Autodesk Fusion 360 part; units mm, degrees
(part 2 of 7)
  spline S350 degree 3 poles (139.4271, 55.7466) (139.3722, 56.1473) (139.3138, 56.5474) (139.2519, 56.9471) knots 0 0 0 0 1 1 1 1
  line L94 (27.4293, 60.8238) -> (26.9565, 60.2606)
  line L95 (20.6334, 52.4497) -> (23.1986, 52.6739)
  spline S351 degree 3 poles (30.486, 54.5663) (30.8444, 54.6152) (31.208, 54.5278) (31.505, 54.3214) knots 0 0 0 0 1 1 1 1
  spline S352 degree 3 poles (5.1253, 21.8055) (5.4629, 21.4735) (5.8386, 21.1826) (6.2446, 20.9389) knots 0 0 0 0 1 1 1 1
  spline S353 degree 3 poles (6.2446, 20.9389) (6.6506, 20.695) (7.0841, 20.5001) (7.536, 20.3581) knots 0 0 0 0 1 1 1 1
  spline S354 degree 3 poles (8.9271, 20.0961) (13.5524, 19.7823) (18.173, 19.4041) (22.7877, 18.9618) knots 0 0 0 0 1 1 1 1
  spline S355 degree 3 poles (11.3218, 69.3267) (11.3217, 69.4797) (11.3016, 69.6321) (11.2618, 69.7799) knots 0 0 0 0 1 1 1 1
  spline S356 degree 3 poles (10.8092, 70.5643) (10.7011, 70.6724) (10.5793, 70.7659) (10.4469, 70.8423) knots 0 0 0 0 1 1 1 1
  spline S357 degree 3 poles (4.2406, 22.9109) (4.4908, 22.5088) (4.7878, 22.1378) (5.1253, 21.8055) knots 0 0 0 0 1 1 1 1
  line L96 (9.4976, 59.2549) -> (9.0248, 58.6917)
  spline S358 degree 3 poles (12.9046, 79.647) (12.757, 79.6866) (12.6048, 79.7068) (12.4519, 79.7069) knots 0 0 0 0 1 1 1 1
  line L97 (9.9358, 53.6718) -> (10.9606, 52.8584)
  spline S359 degree 3 poles (36.6117, 17.4425) (41.2123, 16.872) (45.8047, 16.2375) (50.3876, 15.5393) knots 0 0 0 0 1 1 1 1
  line L98 (6.5164, 57.9904) -> (6.9174, 53.4077)
  line L99 (9.5715, 71.0769) -> (9.5715, 71.0769)
  line L100 (10.9606, 52.8584) -> (12.5548, 52.998)
  spline S360 degree 3 poles (11.2618, 69.7799) (11.2223, 69.9274) (11.1636, 70.0692) (11.0872, 70.2015) knots 0 0 0 0 1 1 1 1
  spline S361 degree 3 poles (12.5548, 52.998) (12.9131, 53.0466) (13.2765, 52.959) (13.5733, 52.7525) knots 0 0 0 0 1 1 1 1
  spline S362 degree 3 poles (10.0247, 71.017) (9.8769, 71.0567) (9.7245, 71.0769) (9.5715, 71.0769) knots 0 0 0 0 1 1 1 1
  spline S363 degree 3 poles (7.536, 20.3581) (7.9877, 20.2162) (8.4547, 20.1282) (8.9271, 20.0961) knots 0 0 0 0 1 1 1 1
  line L101 (12.4519, 79.7069) -> (12.4519, 79.7069)
  spline S364 degree 3 poles (15.2828, 57.8989) (15.1809, 57.9845) (15.1178, 58.1074) (15.1076, 58.24) knots 0 0 0 0 1 1 1 1
  line L102 (15.1076, 58.24) -> (15.0203, 59.2363)
  line L103 (32.4104, 61.2595) -> (27.4293, 60.8238)
  spline S365 degree 3 poles (1.0992, 34.3138) (1.3959, 32.5982) (1.7565, 30.8943) (2.1802, 29.2056) knots 0 0 0 0 1 1 1 1
  spline S366 degree 3 poles (8.3344, 70.5643) (8.0061, 70.2361) (7.8217, 69.7909) (7.8217, 69.3267) knots 0 0 0 0 1 1 1 1
  spline S367 degree 3 poles (10.4469, 70.8423) (10.3144, 70.9188) (10.1725, 70.9775) (10.0247, 71.017) knots 0 0 0 0 1 1 1 1
  spline S368 degree 3 poles (13.3268, 79.4723) (13.1943, 79.5487) (13.0524, 79.6074) (12.9046, 79.647) knots 0 0 0 0 1 1 1 1
  spline S369 degree 3 poles (11.0872, 70.2015) (11.0108, 70.3341) (10.9173, 70.4561) (10.8092, 70.5643) knots 0 0 0 0 1 1 1 1
  spline S370 degree 3 poles (13.5733, 52.7525) (13.8701, 52.5461) (14.0786, 52.236) (14.1578, 51.8833) knots 0 0 0 0 1 1 1 1
  line L104 (23.1986, 52.6739) -> (22.7976, 57.2566)
  line L105 (26.9565, 60.2606) -> (26.9983, 59.7825)
  spline S371 degree 3 poles (13.6891, 79.1943) (13.581, 79.3024) (13.4592, 79.3958) (13.3268, 79.4723) knots 0 0 0 0 1 1 1 1
  spline S372 degree 3 poles (8.3344, 68.0895) (8.6625, 67.7614) (9.1075, 67.577) (9.5715, 67.5769) knots 0 0 0 0 1 1 1 1
  line L106 (6.9174, 53.4077) -> (9.9358, 53.6718)
  line L107 (14.1578, 51.8833) -> (14.241, 50.9366)
  spline S373 degree 3 poles (0.092, 44.7003) (0.1305, 42.9597) (0.2339, 41.2211) (0.402, 39.4882) knots 0 0 0 0 1 1 1 1
  spline S374 degree 3 poles (7.8217, 69.3267) (7.8218, 68.8626) (8.0062, 68.4176) (8.3344, 68.0895) knots 0 0 0 0 1 1 1 1
  line L108 (14.241, 50.9366) -> (20.716, 51.5035)
  spline S375 degree 3 poles (3.6391, 24.1925) (3.7883, 23.743) (3.9902, 23.3129) (4.2406, 22.9109) knots 0 0 0 0 1 1 1 1
  spline S376 degree 3 poles (10.8092, 68.0895) (11.1373, 68.4176) (11.3217, 68.8626) (11.3218, 69.3267) knots 0 0 0 0 1 1 1 1
  line L109 (26.9983, 59.7825) -> (24.4481, 59.5593)
  line L110 (20.2324, 57.0323) -> (20.1321, 58.178)
  line L111 (20.1321, 58.178) -> (15.6492, 57.7858)
  line L112 (9.0248, 58.6917) -> (9.0666, 58.2137)
  spline S377 degree 3 poles (2.1802, 29.2056) (2.604, 27.517) (3.0906, 25.8448) (3.6391, 24.1925) knots 0 0 0 0 1 1 1 1
  spline S378 degree 3 poles (0.402, 39.4882) (0.57, 37.7553) (0.8025, 36.0293) (1.0992, 34.3138) knots 0 0 0 0 1 1 1 1
  spline S379 degree 3 poles (9.5715, 71.0769) (9.1075, 71.0768) (8.6625, 70.8925) (8.3344, 70.5643) knots 0 0 0 0 1 1 1 1
  spline S380 degree 3 poles (9.5715, 67.5769) (10.0357, 67.5769) (10.4809, 67.7613) (10.8092, 68.0895) knots 0 0 0 0 1 1 1 1
  line L113 (14.4787, 59.6911) -> (9.4976, 59.2549)
  line L114 (9.0666, 58.2137) -> (6.5164, 57.9904)
  line L115 (22.7976, 57.2566) -> (20.2324, 57.0323)
  spline S381 degree 3 poles (22.7877, 18.9618) (27.4026, 18.5195) (32.011, 18.013) (36.6117, 17.4425) knots 0 0 0 0 1 1 1 1
  line L116 (15.0203, 59.2363) -> (14.4787, 59.6911)
  line L117 (20.716, 51.5035) -> (20.6334, 52.4497)
  spline S382 degree 3 poles (15.6492, 57.7858) (15.5168, 57.7727) (15.3847, 57.8135) (15.2828, 57.8989) knots 0 0 0 0 1 1 1 1
  line L118 (56.1976, 85.7716) -> (51.7033, 85.536)
  spline S383 degree 3 poles (71.8669, 89.3322) (71.7344, 89.4088) (71.5925, 89.4677) (71.4447, 89.5073) knots 0 0 0 0 1 1 1 1
  line L119 (45.607, 87.2191) -> (45.1151, 86.6729)
  spline S384 degree 3 poles (72.5072, 88.6919) (72.4307, 88.8243) (72.3373, 88.946) (72.2292, 89.0541) knots 0 0 0 0 1 1 1 1
  line L120 (64.5051, 83.8436) -> (67.5349, 83.8436)
  line L121 (68.4852, 82.9434) -> (70.0851, 82.9434)
  line L122 (78.0851, 81.6933) -> (80.6602, 81.6933)
  line L123 (80.6602, 81.6933) -> (80.6602, 86.2936)
  spline S385 degree 3 poles (73.5851, 87.4434) (73.4521, 87.4421) (73.3241, 87.4944) (73.2301, 87.5886) knots 0 0 0 0 1 1 1 1
  line L124 (51.1783, 86.0088) -> (51.1255, 87.0077)
  line L125 (67.585, 89.4438) -> (67.0651, 88.9234)
  line L126 (33.0388, 59.8089) -> (32.952, 60.8052)
  spline S386 degree 3 poles (51.7033, 85.536) (51.5707, 85.5278) (51.4403, 85.5732) (51.3416, 85.6621) knots 0 0 0 0 1 1 1 1
  line L127 (45.1399, 86.1933) -> (42.5834, 86.0595)
  line L128 (50.0073, 79.6893) -> (50.0569, 78.7406)
  spline S387 degree 3 poles (72.6818, 88.2697) (72.6423, 88.4174) (72.5836, 88.5594) (72.5072, 88.6919) knots 0 0 0 0 1 1 1 1
  line L129 (67.0651, 88.4438) -> (64.5051, 88.4438)
  spline S388 degree 3 poles (72.2292, 89.0541) (72.1211, 89.1622) (71.9993, 89.2557) (71.8669, 89.3322) knots 0 0 0 0 1 1 1 1
  line L130 (32.0895, 53.4522) -> (32.1722, 52.5055)
  spline S389 degree 3 poles (49.4533, 80.5782) (49.7427, 80.3617) (49.9404, 80.0445) (50.0073, 79.6893) knots 0 0 0 0 1 1 1 1
  spline S390 degree 3 poles (51.3416, 85.6621) (51.2428, 85.7511) (51.1839, 85.876) (51.1783, 86.0088) knots 0 0 0 0 1 1 1 1
  spline S391 degree 3 poles (70.9915, 86.0667) (71.4557, 86.0667) (71.9009, 86.2511) (72.2292, 86.5794) knots 0 0 0 0 1 1 1 1
  line L131 (24.8491, 54.9766) -> (27.8675, 55.2407)
  spline S392 degree 3 poles (69.7544, 89.0541) (69.4262, 88.726) (69.2418, 88.281) (69.2417, 87.817) knots 0 0 0 0 1 1 1 1
  spline S393 degree 3 poles (72.2292, 86.5794) (72.5574, 86.9076) (72.7418, 87.3528) (72.7418, 87.817) knots 0 0 0 0 1 1 1 1
  line L132 (70.3523, 89.4438) -> (67.585, 89.4438)
  line L133 (50.0569, 78.7406) -> (56.548, 79.0806)
  line L134 (56.2575, 84.6229) -> (56.1976, 85.7716)
  spline S394 degree 3 poles (31.505, 54.3214) (31.8018, 54.115) (32.0104, 53.8049) (32.0895, 53.4522) knots 0 0 0 0 1 1 1 1
  line L135 (27.8675, 55.2407) -> (28.8923, 54.4268)
  line L136 (28.8923, 54.4268) -> (30.486, 54.5663)
  line L137 (56.4983, 80.0294) -> (59.0698, 80.1642)
  spline S395 degree 3 poles (71.4447, 89.5073) (71.2969, 89.5469) (71.1445, 89.5669) (70.9915, 89.5668) knots 0 0 0 0 1 1 1 1
  spline S396 degree 3 poles (72.7418, 87.817) (72.7417, 87.9699) (72.7215, 88.1221) (72.6818, 88.2697) knots 0 0 0 0 1 1 1 1
  spline S397 degree 3 poles (33.2145, 59.4678) (33.1125, 59.5533) (33.0491, 59.6762) (33.0388, 59.8089) knots 0 0 0 0 1 1 1 1
  line L138 (45.1151, 86.6729) -> (45.1399, 86.1933)
  line L139 (38.0638, 59.7464) -> (33.5809, 59.3547)
  line L140 (24.4481, 59.5593) -> (24.8491, 54.9766)
  line L141 (51.1255, 87.0077) -> (50.6, 87.4811)
  line L142 (59.0698, 80.1642) -> (58.8289, 84.7578)
  line L143 (45.8504, 81.6241) -> (46.8462, 80.7751)
  line L144 (32.1722, 52.5055) -> (38.6478, 53.0724)
  line L145 (46.8462, 80.7751) -> (48.4441, 80.8588)
  line L146 (70.9915, 89.5668) -> (70.9915, 89.5668)
  line L147 (50.6, 87.4811) -> (45.607, 87.2191)
  spline S398 degree 3 poles (69.2417, 87.817) (69.2417, 87.3528) (69.4261, 86.9076) (69.7544, 86.5794) knots 0 0 0 0 1 1 1 1
  line L148 (64.5051, 88.4438) -> (64.5051, 83.8436)
  line L149 (67.5349, 83.8436) -> (68.4852, 82.9434)
  line L150 (67.0651, 88.9234) -> (67.0651, 88.4438)
  spline S399 degree 3 poles (69.7544, 86.5794) (70.0825, 86.2512) (70.5275, 86.0668) (70.9915, 86.0667) knots 0 0 0 0 1 1 1 1
  line L151 (38.1635, 58.6012) -> (38.0638, 59.7464)
  line L152 (41.1298, 54.2428) -> (40.7288, 58.8255)
  spline S400 degree 3 poles (48.4441, 80.8588) (48.8037, 80.8949) (49.1639, 80.7948) (49.4533, 80.5782) knots 0 0 0 0 1 1 1 1
  line L153 (38.5646, 54.0186) -> (41.1298, 54.2428)
  line L154 (38.6478, 53.0724) -> (38.5646, 54.0186)
  line L155 (58.8289, 84.7578) -> (56.2575, 84.6229)
  spline S401 degree 3 poles (70.9915, 89.5668) (70.5275, 89.5667) (70.0825, 89.3823) (69.7544, 89.0541) knots 0 0 0 0 1 1 1 1
  line L156 (40.7288, 58.8255) -> (38.1635, 58.6012)
  line L157 (42.5834, 86.0595) -> (42.8242, 81.4655)
  line L158 (42.8242, 81.4655) -> (45.8504, 81.6241)
  spline S402 degree 3 poles (33.5809, 59.3547) (33.4485, 59.3416) (33.3165, 59.3824) (33.2145, 59.4678) knots 0 0 0 0 1 1 1 1
  line L159 (32.952, 60.8052) -> (32.4104, 61.2595)
  line L160 (56.548, 79.0806) -> (56.4983, 80.0294)
  line L161 (78.0851, 86.2936) -> (78.0851, 87.4434)
  line L162 (71.5853, 81.6933) -> (71.5853, 80.7435)
  line L163 (78.0851, 80.7435) -> (78.0851, 81.6933)
  line L164 (80.6602, 86.2936) -> (78.0851, 86.2936)
  spline S403 degree 3 poles (71.6313, 89.4438) (71.7125, 89.4125) (71.7912, 89.3752) (71.8669, 89.3322) knots 0 0 0 0 1 1 1 1
  line L165 (73.0849, 88.9435) -> (72.5852, 89.4438)
  line L166 (73.0849, 87.9436) -> (73.0849, 88.9435)
  spline S404 degree 3 poles (71.8669, 89.3322) (71.9993, 89.2557) (72.1211, 89.1622) (72.2292, 89.0541) knots 0 0 0 0 1 1 1 1
  spline S405 degree 3 poles (72.5072, 88.6919) (72.5836, 88.5594) (72.6423, 88.4174) (72.6818, 88.2697) knots 0 0 0 0 1 1 1 1
  spline S406 degree 3 poles (72.2292, 89.0541) (72.3373, 88.946) (72.4307, 88.8243) (72.5072, 88.6919) knots 0 0 0 0 1 1 1 1
  spline S407 degree 3 poles (70.0851, 82.9434) (70.4462, 82.9607) (70.8006, 82.842) (71.0783, 82.6106) knots 0 0 0 0 1 1 1 1
  spline S408 degree 3 poles (72.6818, 88.2697) (72.7215, 88.1221) (72.7417, 87.9699) (72.7418, 87.817) knots 0 0 0 0 1 1 1 1
  spline S409 degree 3 poles (71.0783, 82.6106) (71.3562, 82.3791) (71.5371, 82.0518) (71.5853, 81.6933) knots 0 0 0 0 1 1 1 1
  spline S410 degree 3 poles (72.2292, 86.5794) (71.9009, 86.2511) (71.4557, 86.0667) (70.9915, 86.0667) knots 0 0 0 0 1 1 1 1
  spline S411 degree 3 poles (74.522, 80.7435) (74.4176, 80.5939) (74.3469, 80.4234) (74.3148, 80.2438) knots 0 0 0 0 1 1 1 1
  spline S412 degree 3 poles (69.7544, 89.0541) (69.9248, 89.2237) (70.1283, 89.3563) (70.3523, 89.4438) knots 0 0 0 0 1 1 1 1
  spline S413 degree 3 poles (69.7544, 86.5794) (69.4261, 86.9076) (69.2417, 87.3528) (69.2417, 87.817) knots 0 0 0 0 1 1 1 1
  line L167 (78.0851, 87.4434) -> (73.5851, 87.4434)
  line L168 (72.5852, 89.4438) -> (71.6313, 89.4438)
  spline S414 degree 3 poles (72.7418, 87.817) (72.7418, 87.3528) (72.5574, 86.9076) (72.2292, 86.5794) knots 0 0 0 0 1 1 1 1
  spline S415 degree 3 poles (70.9915, 86.0667) (70.5275, 86.0668) (70.0825, 86.2512) (69.7544, 86.5794) knots 0 0 0 0 1 1 1 1
  line L169 (71.5853, 80.7435) -> (78.0851, 80.7435)
  spline S416 degree 3 poles (73.2301, 87.5886) (73.136, 87.6826) (73.0836, 87.8106) (73.0849, 87.9436) knots 0 0 0 0 1 1 1 1
  spline S417 degree 3 poles (74.3148, 80.2438) (74.3148, 79.9094) (74.4477, 79.5887) (74.6843, 79.3524) knots 0 0 0 0 1 1 1 1
  spline S418 degree 3 poles (75.5752, 78.9834) (75.9094, 78.9834) (76.2298, 79.1162) (76.4661, 79.3524) knots 0 0 0 0 1 1 1 1
  spline S419 degree 3 poles (76.8351, 80.2438) (76.8351, 80.376) (76.8144, 80.5073) (76.7736, 80.6329) knots 0 0 0 0 1 1 1 1
  spline S420 degree 3 poles (69.2417, 87.817) (69.2418, 88.281) (69.4262, 88.726) (69.7544, 89.0541) knots 0 0 0 0 1 1 1 1
  spline S421 degree 3 poles (74.6843, 79.3524) (74.9206, 79.1162) (75.2411, 78.9834) (75.5752, 78.9834) knots 0 0 0 0 1 1 1 1
  line L170 (70.3523, 89.4438) -> (70.3523, 89.4438)
  spline S422 degree 3 poles (76.4661, 79.3524) (76.7025, 79.5888) (76.8352, 79.9095) (76.8351, 80.2438) knots 0 0 0 0 1 1 1 1
  spline S423 degree 3 poles (76.7736, 80.6329) (76.7566, 80.6707) (76.7378, 80.7076) (76.7173, 80.7435) knots 0 0 0 0 1 1 1 1
  spline S424 degree 3 poles (71.5853, 81.6303) (71.5679, 81.6539) (71.5499, 81.6772) (71.5315, 81.7001) knots 0 0 0 0 1 1 1 1
  line L171 (76.7173, 80.7435) -> (74.522, 80.7435)
  spline S425 degree 3 poles (71.5315, 81.7001) (71.4043, 81.8274) (71.261, 81.9376) (71.1052, 82.0277) knots 0 0 0 0 1 1 1 1
  spline S426 degree 3 poles (70.0753, 82.3036) (69.5289, 82.3036) (69.0048, 82.0865) (68.6185, 81.7001) knots 0 0 0 0 1 1 1 1
  spline S427 degree 3 poles (71.1052, 82.0277) (70.9492, 82.1177) (70.7821, 82.1868) (70.6081, 82.2334) knots 0 0 0 0 1 1 1 1
  spline S428 degree 3 poles (68.6185, 81.7001) (68.2322, 81.3139) (68.0151, 80.7901) (68.0149, 80.2438) knots 0 0 0 0 1 1 1 1
  spline S429 degree 3 poles (68.6185, 78.7871) (69.0048, 78.4006) (69.5289, 78.1835) (70.0753, 78.1835) knots 0 0 0 0 1 1 1 1
  line L172 (72.069, 80.7435) -> (71.5853, 80.7435)
  spline S430 degree 3 poles (68.0149, 80.2438) (68.015, 79.6974) (68.2321, 79.1734) (68.6185, 78.7871) knots 0 0 0 0 1 1 1 1
  spline S431 degree 3 poles (63.315, 80.2438) (63.3148, 79.9095) (63.4476, 79.5888) (63.6839, 79.3524) knots 0 0 0 0 1 1 1 1
  spline S432 degree 3 poles (63.6839, 81.1347) (63.4477, 80.8984) (63.315, 80.578) (63.315, 80.2438) knots 0 0 0 0 1 1 1 1
  spline S433 degree 3 poles (64.9645, 81.4417) (64.8387, 81.4827) (64.7072, 81.5036) (64.5748, 81.5037) knots 0 0 0 0 1 1 1 1
  spline S434 degree 3 poles (71.5315, 78.7871) (71.6589, 78.9143) (71.769, 79.0576) (71.8592, 79.2134) knots 0 0 0 0 1 1 1 1
  spline S435 degree 3 poles (72.1351, 80.2438) (72.1336, 80.4125) (72.1114, 80.5803) (72.069, 80.7435) knots 0 0 0 0 1 1 1 1
  spline S436 degree 3 poles (64.5748, 81.5037) (64.2407, 81.5037) (63.9202, 81.371) (63.6839, 81.1347) knots 0 0 0 0 1 1 1 1
  spline S437 degree 3 poles (65.4663, 79.3524) (65.7026, 79.5888) (65.8354, 79.9095) (65.8352, 80.2438) knots 0 0 0 0 1 1 1 1
  spline S438 degree 3 poles (65.7732, 80.6329) (65.7324, 80.7587) (65.6721, 80.8773) (65.5944, 80.9843) knots 0 0 0 0 1 1 1 1
  line L173 (64.5748, 81.5037) -> (64.5748, 81.5037)
  spline S439 degree 3 poles (65.5944, 80.9843) (65.5168, 81.0912) (65.4228, 81.1852) (65.3159, 81.2629) knots 0 0 0 0 1 1 1 1
  spline S440 degree 3 poles (64.4203, 77.3437) (64.0986, 77.3439) (63.8013, 77.1723) (63.6405, 76.8936) knots 0 0 0 0 1 1 1 1
  line L174 (64.4203, 75.5439) -> (65.7303, 75.5439)
  spline S441 degree 3 poles (63.6405, 75.9934) (63.8015, 75.715) (64.0987, 75.5436) (64.4203, 75.5439) knots 0 0 0 0 1 1 1 1
  spline S442 degree 3 poles (63.6405, 76.8936) (63.4797, 76.6151) (63.4797, 76.272) (63.6405, 75.9934) knots 0 0 0 0 1 1 1 1
  spline S443 degree 3 poles (64.5748, 78.9834) (64.9092, 78.9833) (65.2298, 79.116) (65.4663, 79.3524) knots 0 0 0 0 1 1 1 1
  spline S444 degree 3 poles (70.0753, 78.1835) (70.2552, 78.1835) (70.4343, 78.2072) (70.6081, 78.2538) knots 0 0 0 0 1 1 1 1
  spline S445 degree 3 poles (65.7303, 75.5439) (66.0517, 75.5438) (66.3488, 75.7152) (66.5096, 75.9934) knots 0 0 0 0 1 1 1 1
  spline S446 degree 3 poles (70.6081, 82.2334) (70.4343, 82.28) (70.2552, 82.3036) (70.0753, 82.3036) knots 0 0 0 0 1 1 1 1
  spline S447 degree 3 poles (70.6081, 78.2538) (70.7821, 78.3003) (70.9492, 78.3694) (71.1052, 78.4594) knots 0 0 0 0 1 1 1 1
  spline S448 degree 3 poles (72.0648, 79.7105) (72.1115, 79.8845) (72.1351, 80.0637) (72.1351, 80.2438) knots 0 0 0 0 1 1 1 1
  line L175 (71.5853, 80.7435) -> (71.5853, 81.6303)
  spline S449 degree 3 poles (71.1052, 78.4594) (71.261, 78.5496) (71.4043, 78.6597) (71.5315, 78.7871) knots 0 0 0 0 1 1 1 1
  spline S450 degree 3 poles (63.6839, 79.3524) (63.9202, 79.1162) (64.2407, 78.9834) (64.5748, 78.9834) knots 0 0 0 0 1 1 1 1
  spline S451 degree 3 poles (65.8352, 80.2438) (65.8351, 80.376) (65.8142, 80.5073) (65.7732, 80.6329) knots 0 0 0 0 1 1 1 1
  spline S452 degree 3 poles (65.3159, 81.2629) (65.2089, 81.3406) (65.0903, 81.4009) (64.9645, 81.4417) knots 0 0 0 0 1 1 1 1
  spline S453 degree 3 poles (65.7303, 77.3437) (66.0518, 77.3437) (66.3489, 77.1721) (66.5096, 76.8936) knots 0 0 0 0 1 1 1 1
  line L176 (65.7303, 77.3437) -> (64.4203, 77.3437)
  spline S454 degree 3 poles (66.5096, 75.9934) (66.6705, 76.272) (66.6705, 76.6151) (66.5096, 76.8936) knots 0 0 0 0 1 1 1 1
  spline S455 degree 3 poles (66.5096, 76.8936) (66.3489, 77.1721) (66.0518, 77.3437) (65.7303, 77.3437) knots 0 0 0 0 1 1 1 1
  spline S456 degree 3 poles (71.8592, 79.2134) (71.9492, 79.3694) (72.0183, 79.5365) (72.0648, 79.7105) knots 0 0 0 0 1 1 1 1
  line L177 (65.7303, 75.5439) -> (64.4203, 75.5439)
  spline S457 degree 3 poles (63.6405, 76.8936) (63.8013, 77.1723) (64.0986, 77.3439) (64.4203, 77.3437) knots 0 0 0 0 1 1 1 1
  spline S458 degree 3 poles (66.5096, 76.8936) (66.6705, 76.6151) (66.6705, 76.272) (66.5096, 75.9934) knots 0 0 0 0 1 1 1 1
  spline S459 degree 3 poles (64.4203, 75.5439) (64.0987, 75.5436) (63.8015, 75.715) (63.6405, 75.9934) knots 0 0 0 0 1 1 1 1
  line L178 (64.4203, 77.3437) -> (64.4203, 77.3437)
  line L179 (64.4203, 77.3437) -> (65.7303, 77.3437)
  spline S460 degree 3 poles (66.5096, 75.9934) (66.3488, 75.7152) (66.0517, 75.5438) (65.7303, 75.5439) knots 0 0 0 0 1 1 1 1
  spline S461 degree 3 poles (63.6405, 75.9934) (63.4797, 76.272) (63.4797, 76.6151) (63.6405, 76.8936) knots 0 0 0 0 1 1 1 1
  spline S462 degree 3 poles (11.8272, 44.7525) (11.9628, 45.0438) (12.2434, 45.2408) (12.5636, 45.2692) knots 0 0 0 0 1 1 1 1
  spline S463 degree 3 poles (13.3134, 52.2967) (13.1395, 52.3433) (12.9602, 52.367) (12.7801, 52.367) knots 0 0 0 0 1 1 1 1
  spline S464 degree 3 poles (38.9325, 35.4202) (38.9325, 35.0858) (38.7996, 34.7651) (38.563, 34.5288) knots 0 0 0 0 1 1 1 1
  spline S465 degree 3 poles (38.8705, 35.8093) (38.9114, 35.6837) (38.9324, 35.5524) (38.9325, 35.4202) knots 0 0 0 0 1 1 1 1
  line L180 (7.3008, 51.088) -> (7.3008, 51.088)
  spline S466 degree 3 poles (34.1829, 35.474) (34.2296, 35.3) (34.2532, 35.1207) (34.2532, 34.9407) knots 0 0 0 0 1 1 1 1
  spline S467 degree 3 poles (36.4122, 35.4202) (36.4441, 35.5644) (36.5012, 35.7019) (36.5807, 35.8264) knots 0 0 0 0 1 1 1 1
  spline S468 degree 3 poles (34.1829, 34.4074) (34.1363, 34.2335) (34.0672, 34.0666) (33.9772, 33.9107) knots 0 0 0 0 1 1 1 1
  line L181 (86.2118, 38.372) -> (86.2118, 20.7818)
  spline S469 degree 3 poles (8.5612, 49.8276) (8.5611, 49.9599) (8.5402, 50.0914) (8.4992, 50.2172) knots 0 0 0 0 1 1 1 1
  spline S470 degree 3 poles (7.6905, 51.026) (7.5647, 51.067) (7.4332, 51.0879) (7.3008, 51.088) knots 0 0 0 0 1 1 1 1
  spline S471 degree 3 poles (38.7645, 36.0176) (38.8062, 35.9516) (38.8417, 35.8819) (38.8705, 35.8093) knots 0 0 0 0 1 1 1 1
  spline S472 degree 3 poles (6.4099, 48.9367) (6.6462, 48.7004) (6.9667, 48.5677) (7.3008, 48.5677) knots 0 0 0 0 1 1 1 1
  spline S473 degree 3 poles (8.0414, 48.8085) (8.1484, 48.8862) (8.2426, 48.9802) (8.3204, 49.0871) knots 0 0 0 0 1 1 1 1
  spline S474 degree 3 poles (14.1635, 51.8202) (14.0558, 51.923) (13.9373, 52.0138) (13.81, 52.091) knots 0 0 0 0 1 1 1 1
  spline S475 degree 3 poles (8.3204, 49.0871) (8.3981, 49.1941) (8.4584, 49.3127) (8.4992, 49.4385) knots 0 0 0 0 1 1 1 1
  spline S476 degree 3 poles (12.7801, 52.367) (12.2337, 52.3671) (11.7097, 52.1502) (11.3233, 51.7639) knots 0 0 0 0 1 1 1 1
  line L182 (39.3118, 20.7818) -> (39.3118, 36.0657)
  spline S477 degree 3 poles (11.3233, 51.7639) (10.9371, 51.3775) (10.7202, 50.8535) (10.7203, 50.3072) knots 0 0 0 0 1 1 1 1
  spline S478 degree 3 poles (38.563, 34.5288) (38.3267, 34.2925) (38.0063, 34.1598) (37.6721, 34.1598) knots 0 0 0 0 1 1 1 1
  spline S479 degree 3 poles (34.2532, 34.9407) (34.2532, 34.7606) (34.2296, 34.5813) (34.1829, 34.4074) knots 0 0 0 0 1 1 1 1
  line L183 (36.5807, 35.8264) -> (34.1261, 35.6114)
  spline S480 degree 3 poles (7.3008, 51.088) (6.9666, 51.0879) (6.6462, 50.9549) (6.4099, 50.7185) knots 0 0 0 0 1 1 1 1
  spline S481 degree 3 poles (6.4099, 50.7185) (6.1737, 50.4822) (6.041, 50.1617) (6.041, 49.8276) knots 0 0 0 0 1 1 1 1
  spline S482 degree 3 poles (11.9057, 43.8569) (11.7217, 44.12) (11.6917, 44.4613) (11.8272, 44.7525) knots 0 0 0 0 1 1 1 1
  spline S483 degree 3 poles (7.6905, 48.6292) (7.8161, 48.6702) (7.9345, 48.7307) (8.0414, 48.8085) knots 0 0 0 0 1 1 1 1
  spline S484 degree 3 poles (8.0414, 50.8472) (7.9345, 50.9248) (7.8161, 50.9851) (7.6905, 51.026) knots 0 0 0 0 1 1 1 1
  spline S485 degree 3 poles (13.3134, 48.3171) (13.4872, 48.3638) (13.6542, 48.4332) (13.81, 48.5233) knots 0 0 0 0 1 1 1 1
  spline S486 degree 3 poles (6.041, 49.8276) (6.041, 49.4935) (6.1737, 49.173) (6.4099, 48.9367) knots 0 0 0 0 1 1 1 1
  spline S487 degree 3 poles (14.2369, 48.8504) (14.3641, 48.9778) (14.474, 49.1213) (14.564, 49.2772) knots 0 0 0 0 1 1 1 1
  spline S488 degree 3 poles (14.564, 49.2772) (14.6539, 49.4331) (14.7231, 49.6) (14.7696, 49.7739) knots 0 0 0 0 1 1 1 1
  spline S489 degree 3 poles (12.7801, 48.2473) (12.9601, 48.2472) (13.1394, 48.2706) (13.3134, 48.3171) knots 0 0 0 0 1 1 1 1
  line L184 (52.0955, 38.372) -> (86.2118, 38.372)
  spline S490 degree 3 poles (52.0707, 38.8407) (52.1203, 38.6894) (52.1288, 38.5277) (52.0955, 38.372) knots 0 0 0 0 1 1 1 1
  spline S491 degree 3 poles (14.7696, 49.7739) (14.8163, 49.9478) (14.8399, 50.1271) (14.8399, 50.3072) knots 0 0 0 0 1 1 1 1
  line L185 (39.3118, 36.0657) -> (38.7645, 36.0176)
  spline S492 degree 3 poles (37.6721, 34.1598) (37.338, 34.1598) (37.0175, 34.2925) (36.7812, 34.5288) knots 0 0 0 0 1 1 1 1
  line L186 (12.5636, 45.2692) -> (13.8684, 45.3834)
  spline S493 degree 3 poles (7.3008, 48.5677) (7.4331, 48.5676) (7.5646, 48.5884) (7.6905, 48.6292) knots 0 0 0 0 1 1 1 1
  spline S494 degree 3 poles (34.1261, 35.6114) (34.1467, 35.5663) (34.1656, 35.5204) (34.1829, 35.474) knots 0 0 0 0 1 1 1 1
  spline S495 degree 3 poles (8.4992, 50.2172) (8.4584, 50.3429) (8.398, 50.4613) (8.3204, 50.5681) knots 0 0 0 0 1 1 1 1
  line L187 (86.2118, 20.7818) -> (39.3118, 20.7818)
  spline S496 degree 3 poles (8.3204, 50.5681) (8.2426, 50.6752) (8.1485, 50.7694) (8.0414, 50.8472) knots 0 0 0 0 1 1 1 1
  spline S497 degree 3 poles (11.3233, 48.8504) (11.7097, 48.4642) (12.2337, 48.2472) (12.7801, 48.2473) knots 0 0 0 0 1 1 1 1
  line L188 (13.9469, 45.3865) -> (13.9469, 45.3865)
  spline S498 degree 3 poles (13.81, 52.091) (13.6542, 52.181) (13.4872, 52.2501) (13.3134, 52.2967) knots 0 0 0 0 1 1 1 1
  spline S499 degree 3 poles (14.8399, 50.3072) (14.8399, 50.4872) (14.8163, 50.6665) (14.7696, 50.8405) knots 0 0 0 0 1 1 1 1
  spline S500 degree 3 poles (10.7203, 50.3072) (10.7202, 49.7608) (10.9371, 49.2368) (11.3233, 48.8504) knots 0 0 0 0 1 1 1 1
  spline S501 degree 3 poles (36.7812, 34.5288) (36.5448, 34.7652) (36.4121, 35.0859) (36.4122, 35.4202) knots 0 0 0 0 1 1 1 1
  spline S502 degree 3 poles (13.81, 48.5233) (13.966, 48.6132) (14.1095, 48.7232) (14.2369, 48.8504) knots 0 0 0 0 1 1 1 1
  spline S503 degree 3 poles (8.4992, 49.4385) (8.5402, 49.5641) (8.5611, 49.6954) (8.5612, 49.8276) knots 0 0 0 0 1 1 1 1
  spline S504 degree 3 poles (13.8684, 45.3834) (13.8945, 45.3856) (13.9207, 45.3866) (13.9469, 45.3865) knots 0 0 0 0 1 1 1 1
  spline S505 degree 3 poles (54.0664, 60.5825) (53.8302, 60.8188) (53.6975, 61.1393) (53.6975, 61.4734) knots 0 0 0 0 1 1 1 1
  spline S506 degree 3 poles (43.1286, 59.9872) (43.0811, 59.7425) (42.9933, 59.5075) (42.8687, 59.2916) knots 0 0 0 0 1 1 1 1
  spline S507 degree 3 poles (34.9307, 52.3551) (34.9625, 52.4995) (35.0196, 52.6372) (35.0991, 52.7618) knots 0 0 0 0 1 1 1 1
  spline S508 degree 3 poles (41.8967, 62.4439) (42.0484, 62.3707) (42.1914, 62.2808) (42.323, 62.1757) knots 0 0 0 0 1 1 1 1
  spline S509 degree 3 poles (32.7014, 52.4088) (32.7479, 52.2351) (32.7716, 52.056) (32.7716, 51.8761) knots 0 0 0 0 1 1 1 1
  spline S510 degree 3 poles (32.6445, 52.5468) (32.6651, 52.5015) (32.6841, 52.4555) (32.7014, 52.4088) knots 0 0 0 0 1 1 1 1
  spline S511 degree 3 poles (35.2996, 51.4642) (35.0634, 51.7005) (34.9307, 52.021) (34.9307, 52.3551) knots 0 0 0 0 1 1 1 1
  spline S512 degree 3 poles (42.6795, 61.8196) (42.7768, 61.6971) (42.8609, 61.5648) (42.9307, 61.4248) knots 0 0 0 0 1 1 1 1
  spline S513 degree 3 poles (32.4957, 50.8461) (32.4056, 50.6901) (32.2955, 50.5466) (32.1681, 50.4193) knots 0 0 0 0 1 1 1 1
  spline S514 degree 3 poles (54.9574, 60.2135) (54.6232, 60.2135) (54.3027, 60.3462) (54.0664, 60.5825) knots 0 0 0 0 1 1 1 1
  spline S515 degree 3 poles (32.7014, 51.3428) (32.6548, 51.1689) (32.5856, 51.002) (32.4957, 50.8461) knots 0 0 0 0 1 1 1 1
  spline S516 degree 3 poles (42.8687, 59.2916) (42.6713, 58.9498) (42.3874, 58.6658) (42.0455, 58.4684) knots 0 0 0 0 1 1 1 1
  spline S517 degree 3 poles (44.8634, 61.7886) (45.0997, 61.5523) (45.2324, 61.2319) (45.2324, 60.8977) knots 0 0 0 0 1 1 1 1
  spline S518 degree 3 poles (30.133, 34.9407) (30.1331, 35.4871) (30.3502, 36.0111) (30.7366, 36.3974) knots 0 0 0 0 1 1 1 1
  spline S519 degree 3 poles (43.9725, 62.1576) (44.3066, 62.1576) (44.6271, 62.0249) (44.8634, 61.7886) knots 0 0 0 0 1 1 1 1
  spline S520 degree 3 poles (43.9725, 59.6373) (43.6573, 59.6443) (43.3562, 59.7691) (43.1286, 59.9872) knots 0 0 0 0 1 1 1 1
  spline S521 degree 3 poles (36.1905, 51.0952) (35.8564, 51.0952) (35.5359, 51.2279) (35.2996, 51.4642) knots 0 0 0 0 1 1 1 1
  spline S522 degree 3 poles (37.0814, 51.4642) (36.8451, 51.2279) (36.5247, 51.0952) (36.1905, 51.0952) knots 0 0 0 0 1 1 1 1
  line L189 (38.6478, 53.0724) -> (37.283, 52.953)
  spline S523 degree 3 poles (33.6496, 33.4839) (33.5224, 33.3567) (33.3791, 33.2467) (33.2233, 33.1568) knots 0 0 0 0 1 1 1 1
  spline S524 degree 3 poles (54.0664, 62.3643) (54.3027, 62.6006) (54.6232, 62.7333) (54.9574, 62.7333) knots 0 0 0 0 1 1 1 1
  spline S525 degree 3 poles (42.0455, 58.4684) (41.7035, 58.2708) (41.3155, 58.1667) (40.9205, 58.1666) knots 0 0 0 0 1 1 1 1
  spline S526 degree 3 poles (32.1681, 50.4193) (32.0409, 50.2919) (31.8975, 50.1818) (31.7417, 50.0917) knots 0 0 0 0 1 1 1 1
  spline S527 degree 3 poles (31.7417, 50.0917) (31.5857, 50.0017) (31.4186, 49.9325) (31.2446, 49.886) knots 0 0 0 0 1 1 1 1
  spline S528 degree 3 poles (40.9205, 62.6666) (41.0888, 62.6666) (41.2566, 62.6477) (41.4207, 62.6103) knots 0 0 0 0 1 1 1 1
  spline S529 degree 3 poles (31.2446, 49.886) (31.0708, 49.8394) (30.8917, 49.8158) (30.7118, 49.8157) knots 0 0 0 0 1 1 1 1
  spline S530 degree 3 poles (29.2551, 50.4193) (28.8686, 50.8056) (28.6515, 51.3296) (28.6515, 51.8761) knots 0 0 0 0 1 1 1 1
  spline S531 degree 3 poles (29.2551, 53.3323) (29.6414, 53.7187) (30.1654, 53.9359) (30.7118, 53.9359) knots 0 0 0 0 1 1 1 1
  spline S532 degree 3 poles (31.2446, 53.8656) (31.4186, 53.8191) (31.5857, 53.7499) (31.7417, 53.6599) knots 0 0 0 0 1 1 1 1
  spline S533 degree 3 poles (45.2324, 60.8977) (45.2324, 60.5636) (45.0997, 60.2431) (44.8634, 60.0068) knots 0 0 0 0 1 1 1 1
  spline S534 degree 3 poles (37.283, 52.953) (37.3247, 52.887) (37.3601, 52.8173) (37.3889, 52.7447) knots 0 0 0 0 1 1 1 1
  spline S535 degree 3 poles (32.7262, 32.9506) (32.5524, 32.9042) (32.3733, 32.8807) (32.1934, 32.8808) knots 0 0 0 0 1 1 1 1
  line L190 (32.952, 60.8052) -> (33.0388, 59.8089)
  spline S536 degree 3 poles (31.7417, 53.6599) (31.869, 53.5825) (31.9875, 53.4916) (32.0952, 53.3886) knots 0 0 0 0 1 1 1 1
  spline S537 degree 3 poles (32.7262, 36.9302) (32.9001, 36.8837) (33.0673, 36.8145) (33.2233, 36.7245) knots 0 0 0 0 1 1 1 1
  line L191 (54.9574, 62.7333) -> (54.9574, 62.7333)
  spline S538 degree 3 poles (33.2233, 36.7245) (33.3506, 36.6471) (33.4691, 36.5562) (33.5768, 36.4532) knots 0 0 0 0 1 1 1 1
  line L192 (33.5768, 36.4532) -> (33.5711, 36.5168)
  spline S539 degree 3 poles (42.9307, 61.4248) (42.9616, 61.5532) (43.0125, 61.676) (43.0816, 61.7886) knots 0 0 0 0 1 1 1 1
  spline S540 degree 3 poles (44.8634, 60.0068) (44.6272, 59.7704) (44.3067, 59.6375) (43.9725, 59.6373) knots 0 0 0 0 1 1 1 1
  line L193 (40.783, 58.2033) -> (41.1298, 54.2428)
  line L194 (41.1298, 54.2428) -> (38.5646, 54.0186)
  spline S541 degree 3 poles (37.3889, 52.7447) (37.4297, 52.6189) (37.4505, 52.4874) (37.4504, 52.3551) knots 0 0 0 0 1 1 1 1
  spline S542 degree 3 poles (32.7716, 51.8761) (32.7716, 51.696) (32.748, 51.5167) (32.7014, 51.3428) knots 0 0 0 0 1 1 1 1
  spline S543 degree 3 poles (30.7366, 33.4839) (30.3502, 33.8702) (30.1331, 34.3942) (30.133, 34.9407) knots 0 0 0 0 1 1 1 1
  spline S544 degree 3 poles (42.323, 62.1757) (42.4548, 62.0707) (42.5744, 61.9513) (42.6795, 61.8196) knots 0 0 0 0 1 1 1 1
  spline S545 degree 3 poles (32.1934, 37.0005) (32.3733, 37.0004) (32.5524, 36.9768) (32.7262, 36.9302) knots 0 0 0 0 1 1 1 1
  spline S546 degree 3 poles (33.2233, 33.1568) (33.0673, 33.0666) (32.9002, 32.9973) (32.7262, 32.9506) knots 0 0 0 0 1 1 1 1
  spline S547 degree 3 poles (32.1934, 32.8808) (31.647, 32.8807) (31.123, 33.0977) (30.7366, 33.4839) knots 0 0 0 0 1 1 1 1
  spline S548 degree 3 poles (40.9205, 58.1666) (40.8743, 58.1774) (40.8284, 58.1896) (40.783, 58.2033) knots 0 0 0 0 1 1 1 1
  line L195 (35.0991, 52.7618) -> (32.6445, 52.5468)
  spline S549 degree 3 poles (28.6515, 51.8761) (28.6516, 52.4223) (28.8687, 52.9461) (29.2551, 53.3323) knots 0 0 0 0 1 1 1 1
  spline S550 degree 3 poles (30.7118, 49.8157) (30.1654, 49.8157) (29.6414, 50.0329) (29.2551, 50.4193) knots 0 0 0 0 1 1 1 1
  spline S551 degree 3 poles (33.9772, 33.9107) (33.8872, 33.7548) (33.777, 33.6112) (33.6496, 33.4839) knots 0 0 0 0 1 1 1 1
  line L196 (32.0952, 53.3886) -> (32.0895, 53.4522)
  spline S552 degree 3 poles (43.0816, 61.7886) (43.3179, 62.0249) (43.6384, 62.1576) (43.9725, 62.1576) knots 0 0 0 0 1 1 1 1
  spline S553 degree 3 poles (37.4504, 52.3551) (37.4504, 52.021) (37.3177, 51.7005) (37.0814, 51.4642) knots 0 0 0 0 1 1 1 1
  line L197 (32.4104, 61.2595) -> (32.952, 60.8052)
  line L198 (38.5646, 54.0186) -> (38.6478, 53.0724)
  spline S554 degree 3 poles (30.7118, 53.9359) (30.8917, 53.9358) (31.0708, 53.9122) (31.2446, 53.8656) knots 0 0 0 0 1 1 1 1
  spline S555 degree 3 poles (32.0895, 53.4522) (32.0104, 53.8049) (31.8018, 54.115) (31.505, 54.3214) knots 0 0 0 0 1 1 1 1
  spline S556 degree 3 poles (41.4207, 62.6103) (41.5851, 62.5728) (41.7447, 62.517) (41.8967, 62.4439) knots 0 0 0 0 1 1 1 1
  spline S557 degree 3 poles (30.7366, 36.3974) (31.123, 36.7837) (31.647, 37.0006) (32.1934, 37.0005) knots 0 0 0 0 1 1 1 1
  spline S558 degree 3 poles (53.6975, 61.4734) (53.6975, 61.8075) (53.8302, 62.128) (54.0664, 62.3643) knots 0 0 0 0 1 1 1 1
  line L199 (20.716, 51.5035) -> (19.3513, 51.3841)
  line L200 (24.8491, 54.9766) -> (24.4481, 59.5593)
  line L201 (33.5809, 59.3547) -> (38.0638, 59.7464)
  spline S559 degree 3 poles (55.6979, 62.4925) (55.8049, 62.4148) (55.8991, 62.3208) (55.9769, 62.2139) knots 0 0 0 0 1 1 1 1
  line L202 (20.1321, 58.178) -> (20.2324, 57.0323)
  spline S560 degree 3 poles (19.4577, 51.1758) (19.4985, 51.0502) (19.5192, 50.9188) (19.5192, 50.7867) knots 0 0 0 0 1 1 1 1
  line L203 (24.4481, 59.5593) -> (26.9983, 59.7825)
  spline S561 degree 3 poles (33.0388, 59.8089) (33.0491, 59.6762) (33.1125, 59.5533) (33.2145, 59.4678) knots 0 0 0 0 1 1 1 1
  line L204 (20.2324, 57.0323) -> (22.7976, 57.2566)
  spline S562 degree 3 poles (14.8399, 50.3072) (14.8399, 50.1271) (14.8163, 49.9478) (14.7696, 49.7739) knots 0 0 0 0 1 1 1 1
  line L205 (27.8675, 55.2407) -> (24.8491, 54.9766)
  spline S563 degree 3 poles (39.5418, 58.7216) (39.319, 58.8758) (39.1259, 59.0689) (38.9718, 59.2916) knots 0 0 0 0 1 1 1 1
  line L206 (23.1986, 52.6739) -> (20.6334, 52.4497)
  line L207 (15.6492, 57.7858) -> (20.1321, 58.178)
  line L208 (49.4647, 63.2454) -> (49.4647, 63.2454)
  spline S564 degree 3 poles (38.9718, 61.5416) (39.1693, 61.8837) (39.4534, 62.1678) (39.7955, 62.3653) knots 0 0 0 0 1 1 1 1
  spline S565 degree 3 poles (14.7696, 49.7739) (14.7231, 49.6) (14.6539, 49.4331) (14.564, 49.2772) knots 0 0 0 0 1 1 1 1
  spline S566 degree 3 poles (19.5192, 50.7867) (19.5194, 50.4524) (19.3866, 50.1317) (19.1502, 49.8953) knots 0 0 0 0 1 1 1 1
  spline S567 degree 3 poles (19.3513, 51.3841) (19.3931, 51.3181) (19.4288, 51.2484) (19.4577, 51.1758) knots 0 0 0 0 1 1 1 1
  spline S568 degree 3 poles (55.3465, 62.6718) (55.4723, 62.6308) (55.5909, 62.5703) (55.6979, 62.4925) knots 0 0 0 0 1 1 1 1
  spline S569 degree 3 poles (48.0084, 59.7288) (47.622, 60.1151) (47.4049, 60.6391) (47.4048, 61.1856) knots 0 0 0 0 1 1 1 1
  spline S570 degree 3 poles (48.0084, 62.6423) (48.3947, 63.0284) (48.9185, 63.2454) (49.4647, 63.2454) knots 0 0 0 0 1 1 1 1
  line L209 (26.9983, 59.7825) -> (26.9565, 60.2606)
  spline S571 degree 3 poles (54.9574, 62.7333) (55.0895, 62.7333) (55.2208, 62.7126) (55.3465, 62.6718) knots 0 0 0 0 1 1 1 1
  spline S572 degree 3 poles (47.4048, 61.1856) (47.4049, 61.732) (47.622, 62.256) (48.0084, 62.6423) knots 0 0 0 0 1 1 1 1
  spline S573 degree 3 poles (56.1557, 61.8625) (56.1965, 61.7368) (56.2173, 61.6055) (56.2172, 61.4734) knots 0 0 0 0 1 1 1 1
  spline S574 degree 3 poles (55.8483, 60.5825) (55.612, 60.3462) (55.2915, 60.2135) (54.9574, 60.2135) knots 0 0 0 0 1 1 1 1
  spline S575 degree 3 poles (14.7128, 50.9779) (14.7334, 50.9328) (14.7523, 50.8869) (14.7696, 50.8405) knots 0 0 0 0 1 1 1 1
  spline S576 degree 3 poles (56.2172, 61.4734) (56.2172, 61.1393) (56.0845, 60.8188) (55.8483, 60.5825) knots 0 0 0 0 1 1 1 1
  spline S577 degree 3 poles (10.8092, 70.5643) (10.9173, 70.4561) (11.0108, 70.3341) (11.0872, 70.2015) knots 0 0 0 0 1 1 1 1
  line L210 (27.4293, 60.8238) -> (32.4104, 61.2595)
  spline S578 degree 3 poles (38.9718, 59.2916) (38.7743, 59.6337) (38.6704, 60.0217) (38.6705, 60.4166) knots 0 0 0 0 1 1 1 1
  spline S579 degree 3 poles (31.505, 54.3214) (31.208, 54.5278) (30.8444, 54.6152) (30.486, 54.5663) knots 0 0 0 0 1 1 1 1
  spline S580 degree 3 poles (15.1076, 58.24) (15.1178, 58.1074) (15.1809, 57.9845) (15.2828, 57.8989) knots 0 0 0 0 1 1 1 1
  spline S581 degree 3 poles (19.1502, 49.8953) (18.9139, 49.659) (18.5935, 49.5263) (18.2593, 49.5263) knots 0 0 0 0 1 1 1 1
  line L211 (38.1635, 58.6012) -> (39.5418, 58.7216)
  line L212 (28.8923, 54.4268) -> (27.8675, 55.2407)
  spline S582 degree 3 poles (18.2593, 49.5263) (17.9252, 49.5263) (17.6047, 49.659) (17.3684, 49.8953) knots 0 0 0 0 1 1 1 1
  line L213 (30.486, 54.5663) -> (28.8923, 54.4268)
  line L214 (20.6334, 52.4497) -> (20.716, 51.5035)
  line L215 (15.0203, 59.2363) -> (15.1076, 58.24)
  spline S583 degree 3 poles (16.999, 50.7867) (17.0309, 50.9309) (17.0879, 51.0684) (17.1674, 51.1929) knots 0 0 0 0 1 1 1 1
  line L216 (14.4787, 59.6911) -> (15.0203, 59.2363)
  spline S584 degree 3 poles (17.3684, 49.8953) (17.1319, 50.1316) (16.999, 50.4523) (16.999, 50.7867) knots 0 0 0 0 1 1 1 1
  spline S585 degree 3 poles (33.2145, 59.4678) (33.3165, 59.3824) (33.4485, 59.3416) (33.5809, 59.3547) knots 0 0 0 0 1 1 1 1
  line L217 (38.0638, 59.7464) -> (38.1635, 58.6012)
  line L218 (22.7976, 57.2566) -> (23.1986, 52.6739)
  spline S586 degree 3 poles (15.2828, 57.8989) (15.3847, 57.8135) (15.5168, 57.7727) (15.6492, 57.7858) knots 0 0 0 0 1 1 1 1
  line L219 (17.1674, 51.1929) -> (14.7128, 50.9779)
  spline S587 degree 3 poles (14.2369, 48.8504) (14.1095, 48.7232) (13.966, 48.6132) (13.81, 48.5233) knots 0 0 0 0 1 1 1 1
  spline S588 degree 3 poles (38.6705, 60.4166) (38.6704, 60.8116) (38.7743, 61.1996) (38.9718, 61.5416) knots 0 0 0 0 1 1 1 1
  spline S589 degree 3 poles (13.81, 48.5233) (13.6542, 48.4332) (13.4872, 48.3638) (13.3134, 48.3171) knots 0 0 0 0 1 1 1 1
  spline S590 degree 3 poles (14.564, 49.2772) (14.474, 49.1213) (14.3641, 48.9778) (14.2369, 48.8504) knots 0 0 0 0 1 1 1 1
  spline S591 degree 3 poles (51.2491, 60.1557) (51.159, 59.9997) (51.0488, 59.8561) (50.9214, 59.7288) knots 0 0 0 0 1 1 1 1
  spline S592 degree 3 poles (50.4951, 59.4017) (50.3391, 59.3115) (50.172, 59.2422) (49.998, 59.1955) knots 0 0 0 0 1 1 1 1
  spline S593 degree 3 poles (49.998, 59.1955) (49.824, 59.1489) (49.6447, 59.1252) (49.4647, 59.1252) knots 0 0 0 0 1 1 1 1
  spline S594 degree 3 poles (50.9214, 59.7288) (50.7942, 59.6016) (50.6509, 59.4916) (50.4951, 59.4017) knots 0 0 0 0 1 1 1 1
  spline S595 degree 3 poles (14.7696, 50.8405) (14.8163, 50.6665) (14.8399, 50.4872) (14.8399, 50.3072) knots 0 0 0 0 1 1 1 1
  spline S596 degree 3 poles (49.4647, 59.1252) (48.9184, 59.1254) (48.3946, 59.3425) (48.0084, 59.7288) knots 0 0 0 0 1 1 1 1
  spline S597 degree 3 poles (55.9769, 62.2139) (56.0546, 62.1069) (56.1149, 61.9883) (56.1557, 61.8625) knots 0 0 0 0 1 1 1 1
  spline S598 degree 3 poles (39.7955, 62.3653) (40.1375, 62.5628) (40.5255, 62.6667) (40.9205, 62.6666) knots 0 0 0 0 1 1 1 1
  spline S599 degree 3 poles (10.4469, 70.8423) (10.5793, 70.7659) (10.7011, 70.6724) (10.8092, 70.5643) knots 0 0 0 0 1 1 1 1
  line L220 (40.9205, 62.6666) -> (40.9205, 62.6666)
  line L221 (26.9565, 60.2606) -> (27.4293, 60.8238)
  spline S600 degree 3 poles (11.0872, 70.2015) (11.1636, 70.0692) (11.2223, 69.9274) (11.2618, 69.7799) knots 0 0 0 0 1 1 1 1
  spline S601 degree 3 poles (108.782, 65.514) (108.612, 65.2415) (108.3097, 65.0802) (107.9887, 65.0907) knots 0 0 0 0 1 1 1 1
  spline S602 degree 3 poles (70.0753, 65.3037) (70.2552, 65.3036) (70.4343, 65.28) (70.6081, 65.2334) knots 0 0 0 0 1 1 1 1
  spline S603 degree 3 poles (72.0648, 62.7105) (72.0183, 62.5365) (71.9492, 62.3694) (71.8592, 62.2134) knots 0 0 0 0 1 1 1 1
  spline S604 degree 3 poles (68.6185, 64.7001) (69.0048, 65.0865) (69.5289, 65.3036) (70.0753, 65.3037) knots 0 0 0 0 1 1 1 1
  spline S605 degree 3 poles (65.5944, 63.9844) (65.6721, 63.8773) (65.7324, 63.7587) (65.7732, 63.633) knots 0 0 0 0 1 1 1 1
  spline S606 degree 3 poles (64.5748, 61.9834) (64.2407, 61.9834) (63.9202, 62.1162) (63.6839, 62.3524) knots 0 0 0 0 1 1 1 1
  spline S607 degree 3 poles (63.315, 63.2438) (63.315, 63.578) (63.4477, 63.8984) (63.6839, 64.1347) knots 0 0 0 0 1 1 1 1
  spline S608 degree 3 poles (64.5748, 64.5037) (64.7072, 64.5036) (64.8387, 64.4827) (64.9645, 64.4417) knots 0 0 0 0 1 1 1 1
  line L222 (64.5748, 64.5037) -> (64.5748, 64.5037)
  spline S609 degree 3 poles (70.6081, 61.2538) (70.4343, 61.2072) (70.2552, 61.1836) (70.0753, 61.1835) knots 0 0 0 0 1 1 1 1
  spline S610 degree 3 poles (75.5752, 64.5037) (75.7074, 64.5036) (75.8387, 64.4826) (75.9643, 64.4417) knots 0 0 0 0 1 1 1 1
  spline S611 degree 3 poles (10.8092, 68.0895) (10.4809, 67.7613) (10.0357, 67.5769) (9.5715, 67.5769) knots 0 0 0 0 1 1 1 1
  spline S612 degree 3 poles (71.5315, 64.7001) (71.6589, 64.5729) (71.769, 64.4296) (71.8592, 64.2737) knots 0 0 0 0 1 1 1 1
  spline S613 degree 3 poles (72.0648, 63.7766) (72.1114, 63.6029) (72.135, 63.4237) (72.1351, 63.2438) knots 0 0 0 0 1 1 1 1
  spline S614 degree 3 poles (68.6185, 61.7871) (68.2321, 62.1734) (68.015, 62.6974) (68.0149, 63.2438) knots 0 0 0 0 1 1 1 1
  spline S615 degree 3 poles (9.5715, 67.5769) (9.1075, 67.577) (8.6625, 67.7614) (8.3344, 68.0895) knots 0 0 0 0 1 1 1 1
  spline S616 degree 3 poles (72.1351, 63.2438) (72.1351, 63.0638) (72.1115, 62.8845) (72.0648, 62.7105) knots 0 0 0 0 1 1 1 1
  spline S617 degree 3 poles (68.0149, 63.2438) (68.0151, 63.7901) (68.2322, 64.3139) (68.6185, 64.7001) knots 0 0 0 0 1 1 1 1
  spline S618 degree 3 poles (65.8352, 63.2438) (65.8354, 62.9095) (65.7026, 62.5888) (65.4663, 62.3524) knots 0 0 0 0 1 1 1 1
  spline S619 degree 3 poles (65.4663, 62.3524) (65.2298, 62.116) (64.9092, 61.9833) (64.5748, 61.9834) knots 0 0 0 0 1 1 1 1
  spline S620 degree 3 poles (76.5943, 63.9844) (76.6721, 63.8774) (76.7326, 63.7588) (76.7736, 63.633) knots 0 0 0 0 1 1 1 1
  spline S621 degree 3 poles (76.3157, 64.2629) (76.4226, 64.1852) (76.5166, 64.0912) (76.5943, 63.9844) knots 0 0 0 0 1 1 1 1
  spline S622 degree 3 poles (76.8351, 63.2438) (76.8352, 62.9095) (76.7025, 62.5888) (76.4661, 62.3524) knots 0 0 0 0 1 1 1 1
  spline S623 degree 3 poles (76.7736, 63.633) (76.8144, 63.5073) (76.8351, 63.376) (76.8351, 63.2438) knots 0 0 0 0 1 1 1 1
  spline S624 degree 3 poles (105.918, 65.6137) (105.7674, 65.8974) (105.7795, 66.2399) (105.9496, 66.5124) knots 0 0 0 0 1 1 1 1
  spline S625 degree 3 poles (71.1052, 65.0277) (71.261, 64.9376) (71.4043, 64.8274) (71.5315, 64.7001) knots 0 0 0 0 1 1 1 1
  spline S626 degree 3 poles (106.6798, 65.1367) (106.359, 65.1485) (106.0687, 65.3303) (105.918, 65.6137) knots 0 0 0 0 1 1 1 1
  spline S627 degree 3 poles (63.6839, 64.1347) (63.9202, 64.371) (64.2407, 64.5037) (64.5748, 64.5037) knots 0 0 0 0 1 1 1 1
  spline S628 degree 3 poles (71.8592, 64.2737) (71.9492, 64.1177) (72.0183, 63.9506) (72.0648, 63.7766) knots 0 0 0 0 1 1 1 1
  spline S629 degree 3 poles (71.5315, 61.7871) (71.4043, 61.6597) (71.261, 61.5496) (71.1052, 61.4594) knots 0 0 0 0 1 1 1 1
  line L223 (70.0753, 65.3037) -> (70.0753, 65.3037)
  spline S630 degree 3 poles (75.5752, 61.9834) (75.2411, 61.9834) (74.9206, 62.1162) (74.6843, 62.3524) knots 0 0 0 0 1 1 1 1
  spline S631 degree 3 poles (76.4661, 62.3524) (76.2298, 62.1162) (75.9094, 61.9834) (75.5752, 61.9834) knots 0 0 0 0 1 1 1 1
  line L224 (75.5752, 64.5037) -> (75.5752, 64.5037)
  spline S632 degree 3 poles (74.6843, 62.3524) (74.4477, 62.5887) (74.3148, 62.9094) (74.3148, 63.2438) knots 0 0 0 0 1 1 1 1
  spline S633 degree 3 poles (74.6843, 64.1347) (74.9206, 64.371) (75.2411, 64.5037) (75.5752, 64.5037) knots 0 0 0 0 1 1 1 1
  spline S634 degree 3 poles (74.3148, 63.2438) (74.3149, 63.578) (74.4479, 63.8985) (74.6843, 64.1347) knots 0 0 0 0 1 1 1 1
  spline S635 degree 3 poles (49.4647, 63.2454) (49.6447, 63.2454) (49.824, 63.2217) (49.998, 63.1751) knots 0 0 0 0 1 1 1 1
  spline S636 degree 3 poles (8.3344, 68.0895) (8.0062, 68.4176) (7.8218, 68.8626) (7.8217, 69.3267) knots 0 0 0 0 1 1 1 1
  spline S637 degree 3 poles (11.2618, 69.7799) (11.3016, 69.6321) (11.3217, 69.4797) (11.3218, 69.3267) knots 0 0 0 0 1 1 1 1
  spline S638 degree 3 poles (108.813, 66.4121) (108.9635, 66.1286) (108.9517, 65.7864) (108.782, 65.514) knots 0 0 0 0 1 1 1 1
  line L225 (107.9887, 65.0907) -> (106.6798, 65.1367)
  spline S639 degree 3 poles (70.6081, 65.2334) (70.7821, 65.1868) (70.9492, 65.1177) (71.1052, 65.0277) knots 0 0 0 0 1 1 1 1
  spline S640 degree 3 poles (70.0753, 61.1835) (69.5289, 61.1835) (69.0048, 61.4006) (68.6185, 61.7871) knots 0 0 0 0 1 1 1 1
  spline S641 degree 3 poles (71.8592, 62.2134) (71.769, 62.0576) (71.6589, 61.9143) (71.5315, 61.7871) knots 0 0 0 0 1 1 1 1
  spline S642 degree 3 poles (64.9645, 64.4417) (65.0903, 64.4009) (65.2089, 64.3406) (65.3159, 64.2629) knots 0 0 0 0 1 1 1 1
  spline S643 degree 3 poles (71.1052, 61.4594) (70.9492, 61.3695) (70.7821, 61.3003) (70.6081, 61.2538) knots 0 0 0 0 1 1 1 1
  spline S644 degree 3 poles (65.7732, 63.633) (65.8142, 63.5073) (65.8351, 63.376) (65.8352, 63.2438) knots 0 0 0 0 1 1 1 1
  spline S645 degree 3 poles (63.6839, 62.3524) (63.4476, 62.5888) (63.3148, 62.9095) (63.315, 63.2438) knots 0 0 0 0 1 1 1 1
  spline S646 degree 3 poles (75.9643, 64.4417) (76.0901, 64.4009) (76.2087, 64.3406) (76.3157, 64.2629) knots 0 0 0 0 1 1 1 1
  spline S647 degree 3 poles (8.3344, 70.5643) (8.6625, 70.8925) (9.1075, 71.0768) (9.5715, 71.0769) knots 0 0 0 0 1 1 1 1
  spline S648 degree 3 poles (105.9496, 66.5124) (106.1195, 66.7849) (106.4218, 66.9462) (106.7428, 66.9356) knots 0 0 0 0 1 1 1 1
  spline S649 degree 3 poles (11.3218, 69.3267) (11.3217, 68.8626) (11.1373, 68.4176) (10.8092, 68.0895) knots 0 0 0 0 1 1 1 1
  spline S650 degree 3 poles (65.3159, 64.2629) (65.4228, 64.1852) (65.5168, 64.0912) (65.5944, 63.9844) knots 0 0 0 0 1 1 1 1
  line L226 (106.7428, 66.9356) -> (106.7428, 66.9356)
  spline S651 degree 3 poles (7.8217, 69.3267) (7.8217, 69.7909) (8.0061, 70.2361) (8.3344, 70.5643) knots 0 0 0 0 1 1 1 1
  line L227 (106.7428, 66.9356) -> (108.0518, 66.8896)
  spline S652 degree 3 poles (108.0518, 66.8896) (108.3725, 66.8775) (108.6625, 66.6956) (108.813, 66.4121) knots 0 0 0 0 1 1 1 1
  line L228 (9.5715, 71.0769) -> (9.5715, 71.0769)
  spline S653 degree 3 poles (107.9887, 65.0907) (108.3097, 65.0802) (108.612, 65.2415) (108.782, 65.514) knots 0 0 0 0 1 1 1 1
  spline S654 degree 3 poles (112.4748, 55.9879) (112.1406, 55.988) (111.8201, 55.8552) (111.5839, 55.619) knots 0 0 0 0 1 1 1 1
  spline S655 degree 3 poles (44.4665, 75.039) (44.7599, 75.0289) (45.0299, 74.8763) (45.19, 74.6302) knots 0 0 0 0 1 1 1 1
  spline S656 degree 3 poles (113.7351, 54.7281) (113.735, 54.8602) (113.7141, 54.9915) (113.6731, 55.1172) knots 0 0 0 0 1 1 1 1
  line L229 (70.73, 73.4437) -> (69.42, 73.4437)
  spline S657 degree 3 poles (69.42, 73.4437) (69.0985, 73.4438) (68.8015, 73.6154) (68.6407, 73.8938) knots 0 0 0 0 1 1 1 1
  spline S658 degree 3 poles (84.4734, 74.4147) (84.7943, 74.4083) (85.0874, 74.2315) (85.2428, 73.9507) knots 0 0 0 0 1 1 1 1
  line L230 (84.4418, 72.6148) -> (83.1324, 72.6381)
  spline S659 degree 3 poles (9.5715, 71.0769) (9.7245, 71.0769) (9.8769, 71.0567) (10.0247, 71.017) knots 0 0 0 0 1 1 1 1
  spline S660 degree 3 poles (113.3662, 53.8372) (113.6024, 54.0735) (113.7351, 54.3939) (113.7351, 54.7281) knots 0 0 0 0 1 1 1 1
  line L231 (83.1639, 74.4375) -> (84.4734, 74.4147)
  spline S661 degree 3 poles (106.9784, 56.9801) (106.432, 56.9801) (105.908, 56.763) (105.5217, 56.3766) knots 0 0 0 0 1 1 1 1
  spline S662 degree 3 poles (85.2428, 73.9507) (85.3983, 73.6698) (85.3924, 73.3274) (85.2273, 73.052) knots 0 0 0 0 1 1 1 1
  spline S663 degree 3 poles (71.5093, 74.7935) (71.67, 74.5151) (71.67, 74.1722) (71.5093, 73.8938) knots 0 0 0 0 1 1 1 1
  spline S664 degree 3 poles (45.19, 74.6302) (45.365, 74.3606) (45.383, 74.018) (45.237, 73.7316) knots 0 0 0 0 1 1 1 1
  spline S665 degree 3 poles (82.3608, 73.1016) (82.2051, 73.3829) (82.2112, 73.7258) (82.3769, 74.0013) knots 0 0 0 0 1 1 1 1
  spline S666 degree 3 poles (112.8644, 55.9265) (112.7385, 55.9673) (112.6071, 55.988) (112.4748, 55.9879) knots 0 0 0 0 1 1 1 1
  spline S667 degree 3 poles (105.5217, 53.463) (105.9081, 53.0768) (106.4321, 52.8599) (106.9784, 52.86) knots 0 0 0 0 1 1 1 1
  spline S668 degree 3 poles (42.1917, 78.7654) (42.428, 79.0016) (42.7485, 79.1343) (43.0826, 79.1343) knots 0 0 0 0 1 1 1 1
  spline S669 degree 3 poles (71.5093, 73.8938) (71.3486, 73.6154) (71.0515, 73.4438) (70.73, 73.4437) knots 0 0 0 0 1 1 1 1
  spline S670 degree 3 poles (112.4748, 53.4677) (112.8091, 53.4677) (113.1298, 53.6006) (113.3662, 53.8372) knots 0 0 0 0 1 1 1 1
  spline S671 degree 3 poles (105.5217, 56.3766) (105.1353, 55.9902) (104.9181, 55.4662) (104.9181, 54.9198) knots 0 0 0 0 1 1 1 1
  spline S672 degree 3 poles (104.9181, 54.9198) (104.9181, 54.3734) (105.1353, 53.8494) (105.5217, 53.463) knots 0 0 0 0 1 1 1 1
  spline S673 degree 3 poles (108.0084, 53.1359) (108.1643, 53.2258) (108.3078, 53.3358) (108.4352, 53.463) knots 0 0 0 0 1 1 1 1
  line L232 (44.482, 73.2412) -> (43.1741, 73.1724)
  spline S674 degree 3 poles (106.9784, 52.86) (107.1585, 52.86) (107.3378, 52.8836) (107.5118, 52.9303) knots 0 0 0 0 1 1 1 1
  spline S675 degree 3 poles (107.5118, 52.9303) (107.6856, 52.9768) (107.8525, 53.046) (108.0084, 53.1359) knots 0 0 0 0 1 1 1 1
  spline S676 degree 3 poles (111.2149, 54.7281) (111.2149, 54.3939) (111.3476, 54.0735) (111.5839, 53.8372) knots 0 0 0 0 1 1 1 1
  spline S677 degree 3 poles (108.7623, 53.8899) (108.8523, 54.0457) (108.9214, 54.2127) (108.968, 54.3865) knots 0 0 0 0 1 1 1 1
  spline S678 degree 3 poles (108.4352, 53.463) (108.5624, 53.5904) (108.6724, 53.7339) (108.7623, 53.8899) knots 0 0 0 0 1 1 1 1
  spline S679 degree 3 poles (85.2273, 73.052) (85.0622, 72.7766) (84.7629, 72.61) (84.4418, 72.6148) knots 0 0 0 0 1 1 1 1
  spline S680 degree 3 poles (50.4951, 62.9694) (50.6509, 62.8795) (50.7942, 62.7695) (50.9214, 62.6423) knots 0 0 0 0 1 1 1 1
  spline S681 degree 3 poles (10.0247, 71.017) (10.1725, 70.9775) (10.3144, 70.9188) (10.4469, 70.8423) knots 0 0 0 0 1 1 1 1
  spline S682 degree 3 poles (68.6407, 74.7935) (68.8015, 75.072) (69.0985, 75.2435) (69.42, 75.2436) knots 0 0 0 0 1 1 1 1
  spline S683 degree 3 poles (44.388, 75.0385) (44.4141, 75.0398) (44.4403, 75.0399) (44.4665, 75.039) knots 0 0 0 0 1 1 1 1
  spline S684 degree 3 poles (50.9214, 62.6423) (51.0488, 62.515) (51.159, 62.3715) (51.2491, 62.2155) knots 0 0 0 0 1 1 1 1
  line L233 (69.42, 75.2436) -> (70.73, 75.2436)
  spline S685 degree 3 poles (108.813, 66.4121) (108.6625, 66.6956) (108.3725, 66.8775) (108.0518, 66.8896) knots 0 0 0 0 1 1 1 1
  spline S686 degree 3 poles (113.2158, 55.7471) (113.1088, 55.825) (112.9902, 55.8855) (112.8644, 55.9265) knots 0 0 0 0 1 1 1 1
  line L234 (83.1639, 74.4375) -> (83.1639, 74.4375)